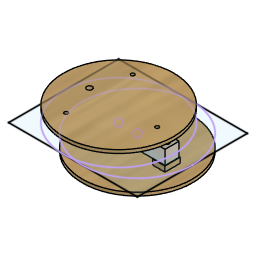
Sensor+de+peso (Autodesk Fusion 360 design; units mm, degrees)
Autodesk Fusion 360 part; units mm, degrees
sketch "Boceto1" plane through (0, 0, 0) normal (0, 0, 1) x (1, 0, 0)
  circle A0 centre (8.5, 0) radius 50
  circle A1 centre (-8.5, 0) radius 50
  line L0 (-8.5, 0) -> (8.5, 0) construction
  line L1 (-40, 6.4) -> (40, 6.4)
  line L2 (40, 6.4) -> (40, -6.4)
  line L3 (40, -6.4) -> (-40, -6.4)
  line L4 (-40, -6.4) -> (-40, 6.4)
  dimension "d1" = 100
  dimension "d2" = 100
  dimension "d3" = 17
  dimension "d8" = 12.8
  dimension "d9" = 80
  dimension "d10" = 6.4
  dimension "d11" = 40
  constraint horizontal A0.centre A1.centre
  constraint coincident A1.centre L0.start
  constraint coincident A0.centre L0.end
  constraint midpoint origin L0
  constraint horizontal L1
  constraint vertical L2
  constraint horizontal L3
  constraint vertical L4
  measures "d1" diameter of A1
  measures "d2" diameter of A0
  measures "d3" distance of A0.centre A1.centre
  measures "d8" distance of L1.start L3.end
  measures "d9" distance of L2.end L3.end
  measures "d10" distance of origin L3
  measures "d11" distance of origin L2
extrude "Extruir1" add sketch "Boceto1" along normal blind 14 contours A0 A1 | A0 A1 | L1 L2 L3 L4 picked at (11.2877, 13.1196) picked at (-47.0762, 0) makes body 1
extrude "Extruir2" add sketch "Boceto1" against normal blind 14 contours A0 A1 | A0 A1 | L1 L2 L3 L4 picked at (51.7978, -9.5063) picked at (11.2877, 13.1196) bodies 1
sketch "Boceto2" plane through (0, 0, 0) normal (0, 1, 0) x (1, 0, 0)
  line L0 (105.3429, 11) -> (-105.3429, 11)
  line L1 (-105.3429, 11) -> (-105.3429, -11)
  line L2 (-105.3429, -11) -> (105.3429, -11)
  line L3 (105.3429, -11) -> (105.3429, 11)
  line L4 (105.3429, 11) -> (-105.3429, -11) construction
  line L5 (-105.3429, 11) -> (105.3429, -11) construction
  dimension "d12" = 22
  constraint horizontal L0
  constraint perpendicular L0 L1
  constraint parallel L0 L2
  constraint parallel L1 L3
  constraint coincident L4 origin
  constraint coincident L5 origin
  measures "d12" distance of L0.end L1.end
extrude "Extruir3" cut sketch "Boceto2" along normal mid plane 120 bodies 1 makes body 2 at (-4.2718, -3.9396, -11)
sketch "Boceto3" plane through (0, 0, 0) normal (0, 1, 0) x (1, 0, 0)
  line L0 (40, 6.35) -> (-40, 6.35)
  line L1 (-40, 6.35) -> (-40, -6.35)
  line L2 (-40, -6.35) -> (40, -6.35)
  line L3 (40, -6.35) -> (40, 6.35)
  line L4 (40, 6.35) -> (-40, -6.35) construction
  line L5 (-40, 6.35) -> (40, -6.35) construction
  circle A0 centre (-3.5, 0) radius 5.5
  circle A1 centre (3.5, 0) radius 5.5
  dimension "d15" = 80
  dimension "d16" = 12.7
  dimension "d17" = 11
  dimension "d18" = 7
  dimension "d19" = 3.5
  constraint horizontal L0
  constraint perpendicular L0 L1
  constraint parallel L0 L2
  constraint parallel L1 L3
  constraint coincident L4 origin
  constraint coincident L5 origin
  constraint equal A0 A1
  constraint horizontal origin A1.centre
  constraint horizontal origin A0.centre
  measures "d15" distance of L1.end L2.end
  measures "d16" distance of L0.start L2.end
  measures "d17" diameter of A0
  measures "d18" distance of A0.centre A1.centre
  measures "d19" distance of origin A1.centre
extrude "Extruir1'" add sketch "Boceto3" along normal mid plane 12.7 separate body makes body 3 in component "Component"
sketch "Boceto4" plane through (0, 0, 0) normal (0, 0, 1) x (1, 0, 0)
  circle A0 centre (35, 0) radius 2.5
  circle A1 centre (-35, 0) radius 2.5
  dimension "d22" = 35
  dimension "d23" = 35
  dimension "d40" = 5
  dimension "d41" = 5
  constraint horizontal origin A1.centre
  constraint horizontal origin A0.centre
  measures "d22" distance of origin A0.centre
  measures "d23" distance of origin A1.centre
  measures "d40" diameter of A1
  measures "d41" diameter of A0
extrude "Extruir4" cut sketch "Boceto4" along normal blind -25 and the other way blind -8 contours A0 bodies 2
extrude "Extruir2'" cut sketch "Boceto4" along normal blind -25 and the other way blind -8 contours A0 bodies 3 in component "Component"
extrude "Extruir5" cut sketch "Boceto4" along normal blind 15 and the other way blind 7 contours A1 bodies 1
extrude "Extruir3'" cut sketch "Boceto4" along normal blind 15 and the other way blind 7 contours A1 bodies 3 in component "Component"
sketch "Boceto5" plane through (0, 0, 14) normal (0, 0, 1) x (-1, 0, 0)
  circle A0 centre (35, 0) radius 2.5
  circle A1 centre (8.5, 0) radius 50
  line L0 (8.5, 0) -> (26, 30.3109) construction
  line L1 (26, -30.3109) -> (8.5, 0) construction
  line L2 (8.5, 0) -> (-26.5, 0) construction
  circle A2 centre (26, 30.3109) radius 1.6
  circle A3 centre (26, -30.3109) radius 1.6
  circle A4 centre (-26.5, 0) radius 1.6
  line L3 (-26.5, 0) -> (26, 30.3109) construction
  line L4 (26, -30.3109) -> (-26.5, 0) construction
  line L5 (26, 30.3109) -> (26, -30.3109) construction
  dimension "d42" = 3.2
  dimension "d43" = 35
  constraint coincident A1.centre L0.start
  constraint equal A2 A3
  constraint equal A3 A4
  constraint equal L0 L2
  constraint equal L0 L1
  constraint equal L3 L5
  constraint equal L4 L5
  constraint horizontal L2
  constraint coincident L0.end A2.centre
  constraint coincident L1.start A3.centre
  constraint coincident L2.end A4.centre
  measures "d42" diameter of A2
  measures "d43" distance of A1.centre L2.end
extrude "Extruir6" cut sketch "Boceto5" against normal blind 6 contours A2 | A3 | A4 bodies 1
extrude "Extruir4'" [no effect] in component "Component"
sketch "Boceto6" plane through (0, 0, 11) normal (0, 0, -1) x (1, 0, 0)
  circle A0 centre (26.5, 0) radius 1.6
  circle A1 centre (-26, -30.3109) radius 1.6
  circle A2 centre (-26, 30.3109) radius 1.6
  circle A3 centre (-35, 0) radius 2.5
  circle A4 centre (-8.5, 0) radius 50
  line L0 (-29.5, -7) -> (-40.5, -7)
  line L1 (-40.5, -7) -> (-40.5, 7)
  line L2 (-40.5, 7) -> (-29.5, 7)
  line L3 (-29.5, 7) -> (-29.5, -7)
  line L4 (-29.5, -7) -> (-40.5, 7) construction
  line L5 (-40.5, -7) -> (-29.5, 7) construction
  point P0 (-35, 0)
  dimension "d48" = 11
  dimension "d49" = 14
  constraint horizontal L0
  constraint perpendicular L0 L1
  constraint parallel L0 L2
  constraint parallel L1 L3
  constraint coincident L4 P0
  constraint coincident L5 P0
  constraint coincident P0 A3.centre
  measures "d48" distance of L1.end L2.end
  measures "d49" distance of L0.start L2.end
extrude "Extruir7" add sketch "Boceto6" along normal blind 4.7 contours L0 L1 L2 L3 bodies 1
sketch "Boceto7" plane through (0, 0, -11) normal (0, 0, 1) x (-1, 0, 0)
  circle A0 centre (-35, 0) radius 2.5
  circle A1 centre (-8.5, 0) radius 50
  line L0 (-29.5, -7) -> (-40.5, -7)
  line L1 (-40.5, -7) -> (-40.5, 7)
  line L2 (-40.5, 7) -> (-29.5, 7)
  line L3 (-29.5, 7) -> (-29.5, -7)
  line L4 (-29.5, -7) -> (-40.5, 7) construction
  line L5 (-40.5, -7) -> (-29.5, 7) construction
  point P0 (-35, 0)
  dimension "d52" = 11
  dimension "d53" = 14
  constraint horizontal L0
  constraint perpendicular L0 L1
  constraint parallel L0 L2
  constraint parallel L1 L3
  constraint coincident L4 P0
  constraint coincident L5 P0
  constraint coincident P0 A0.centre
  measures "d52" distance of L1.end L2.end
  measures "d53" distance of L0.start L2.end
extrude "Extruir8" add sketch "Boceto7" along normal blind 4.77 contours L0 L1 L2 L3 bodies 2
sketch "Boceto8" plane through (0, 0, 0) normal (0, 0, 1) x (1, 0, 0)
  line L0 (58.5, -50) -> (-58.5, -50)
  line L1 (-58.5, -50) -> (-58.5, 50)
  line L2 (-58.5, 50) -> (58.5, 50)
  line L3 (58.5, 50) -> (58.5, -50)
  circle A0 centre (-8.5, 0) radius 50
  circle A1 centre (8.5, 0) radius 50
  dimension "d56" = 117
  dimension "d57" = 100
  constraint horizontal L0
  constraint vertical L1
  constraint horizontal L2
  constraint vertical L3
  constraint tangent L0 A0
  constraint tangent L1 A0
  constraint tangent L2 A0
  constraint tangent L3 A1
  measures "d56" distance of L0.start L0.end
  measures "d57" distance of L0.end L1.end
component "Component" placed x (1, 0, 0) y (0, 1, 0) z (0, 0, 1) at (0, 0, 0)
equation "d10 = d8 / 2"
equation "d19 = d18 / 2"
equation "d23 = d22"
